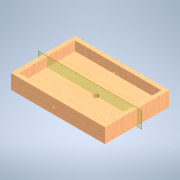
# Autodesk Inventor part: basefresh
Saved by Autodesk Inventor 2020 (Build 240168000, 168)
## iProperties
Created: 2020-05-20
Part Number: basefresh
Material: Wood (Cherry)
Document SubType Name: Modeling
Designer: Manish
Density: 0.63 g/cm^3
Appearance: Cherry - Natural Low Gloss
Author: Manish
Autodesk Inventor part; units mm, degrees
ref_plane "YZ Plane" through (0, 0, 0) normal (1, 0, 0) x (0, 1, 0)
ref_plane "XZ Plane" through (0, 0, 0) normal (0, 1, 0) x (-1, 0, 0)
ref_plane "XY Plane" through (0, 0, 0) normal (0, 0, 1) x (1, 0, 0)
sketch "Sketch1" plane through (0, 0, 0) normal (1, 0, 0) x (0, 1, 0)
  line L0 (0, 0) -> (55, 0)
  line L1 (55, 0) -> (55, -242)
  line L2 (55, -242) -> (0, -242)
  line L3 (0, -242) -> (0, 0)
  dimension "d0" = 55
  dimension "d1" = 242
  constraints: 8 end point, 2 parallel, 1 horizontal, 1 perpendicular
  measures "d0" distance of L1.end L2.end
  measures "d1" distance of L0.end L1.end
extrude "Extrusion1" add sketch "Sketch1" along normal blind 355
sketch "Sketch3" plane through (0, 55, 0) normal (0, 1, 0) x (1, 0, 0)
  circle A0 centre (200, 120) radius 10
  point P0 (0, 0)
  point P1 (0, 0)
  dimension "d8" = 20
  constraints: 1 centre point
  measures "d8" diameter of A0
extrude "Extrusion3" cut sketch "Sketch3" against normal through all
sketch "Sketch4" plane through (0, 55, 0) normal (0, 1, 0) x (1, 0, 0)
  line L0 (15, 15) -> (340, 15)
  line L1 (340, 15) -> (340, 227)
  line L2 (340, 227) -> (15, 227)
  line L3 (15, 227) -> (15, 15)
  line L4 (355, 242) -> (355, 0)
  line L5 (0, 242) -> (355, 242)
  point P0 (0, 0)
  point P1 (0, 0)
  dimension "d11" = 15
  dimension "d12" = 15
  constraints: 12 end point, 2 parallel, 1 horizontal, 1 perpendicular
  measures "d11" distance between parallel lines of L1 L4
  measures "d12" distance between parallel lines of L2 L5
extrude "Extrusion4" cut sketch "Sketch4" against normal blind 35
sketch "Sketch5" plane through (0, 0, 0) normal (0, 0, 1) x (1, 0, 0)
  circle A0 centre (161.4027, 23.0942) radius 3
  line L0 (0, 55) -> (0, 0) projected
  line L1 (355, 55) -> (355, 0) projected
  line L2 (0, 0) -> (355, 0) projected
  dimension "d15" = 6
  dimension "d18" = 161.4027
  dimension "d19" = 355
  dimension "d20" = 23.0942
  constraints: 2 coincident, 1 centre point
  measures "d15" diameter of A0
  measures "d18" distance from line of point (161.403, 23.094) L0
  measures "d19" distance between parallel lines of L1 L0
  measures "d20" distance from line of L2 point (161.403, 23.094)
extrude "Extrusion5" cut sketch "Sketch5" against normal through all
ref_plane "Work Plane1" through (0, 0, -121) normal (0, 0, -1) x (-1, 0, 0)
body "Solid1"
